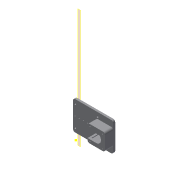
# Autodesk Inventor part: Neje_slide_y_20mmrod_upperplate
Saved by Autodesk Inventor 2019.4 (Build 234330000, 330)
## iProperties
Created: 2021-08-20
Part Number: Neje_slide_y_20mmrod_upperplate
Material: Generic
Document SubType Name: Modeling
Designer: diederichbenedict
Density: 1 g/cm^3
Appearance: Default
Mass: 53.3418 g
Surface Area: 231.662 cm^2
Volume: 53.3418 cm^3
Author: diederichbenedict
Autodesk Inventor part; units mm, degrees
ref_plane "YZ Plane" through (0, 0, 0) normal (1, 0, 0) x (0, 1, 0)
ref_plane "XZ Plane" through (0, 0, 0) normal (0, 1, 0) x (-1, 0, 0)
ref_plane "XY Plane" through (0, 0, 0) normal (0, 0, 1) x (1, 0, 0)
ref_plane "Work Plane1" through (0, 0, 0) normal (0, 0, 1) x (1, 0, 0)
sketch "Sketch1" plane through (0, 0, 0) normal (0, 0, 1) x (1, 0, 0)
  line L0 (40, 0) -> (34, 0) projected
  line L1 (40, 0) -> (40, 260) projected
  line L2 (40, 260) -> (34, 260) projected
  line L3 (34, 0) -> (34, 260) projected
  line L4 (0, 0) -> (6, 0) projected
  line L5 (6, 0) -> (6, 260) projected
  line L6 (0, 260) -> (6, 260) projected
  line L7 (0, 0) -> (0, 260) projected
  line L8 (90, 15.4736) -> (-7, 15.4736)
  line L9 (-7, 15.4736) -> (-7, 85.4736)
  line L10 (-7, 85.4736) -> (90, 85.4736)
  line L11 (90, 85.4736) -> (90, 15.4736)
  line L12 (90, 85.4736) -> (-7, 15.4736) construction
  line L13 (90, 15.4736) -> (-7, 85.4736) construction
  line L14 (14, 0) -> (26, 0) construction
  line L15 (26, 0) -> (26, 260) construction
  line L16 (14, 260) -> (26, 260) construction
  line L17 (14, 0) -> (14, 260) construction
  circle A0 centre (-2, 25.4736) radius 2.45
  circle A1 centre (-2, 75.4736) radius 2.45
  circle A2 centre (51.5, 75.4736) radius 2.45
  circle A3 centre (51.5, 25.4736) radius 2.45
  line L18 (40, 40.4736) -> (-160, 40.4736) projected
  line L19 (40, 60.4736) -> (-160, 60.4736) projected
  circle A4 centre (-2, 25.4736) radius 2.45 construction
  circle A5 centre (-2, 75.4736) radius 2.45 construction
  line L20 (-7, 67.4547) -> (-7, 33.4924) projected
  dimension "d0" = 50
  dimension "d2" = 70
  dimension "d3" = 4.9
  dimension "d4" = 4.9
  dimension "d5" = 4.9
  dimension "d6" = 4.9
  dimension "d7" = 10
  dimension "d10" = 10
  dimension "d11" = 11.5
  dimension "d17" = 25
  dimension "d20" = 0
  constraints: 12 end point, 4 centre point, 2 coincident, 2 parallel, 1 horizontal, 1 perpendicular, 1 point on line
  measures "d0" distance between parallel lines of L11 L1
  measures "d2" distance between parallel lines of L10 L8
  measures "d3" diameter of A0
  measures "d4" diameter of A1
  measures "d5" diameter of A2
  measures "d6" diameter of A3
  measures "d7" distance from line of A3.centre L8
  measures "d10" distance from line of A2.centre L10
  measures "d11" distance from line of L1 A2.centre
  measures "d17" distance between parallel lines of L18 L8
  measures "d20" horizontal distance of A2.centre A3.centre
extrude "Extrusion1" add sketch "Sketch1" along normal blind 5 contours L8 L3 L18 L1 | L1 L10 L11 L8 | L8 L5 L18 L3 | L18 L3 L19 L1 | L18 L5 L19 L3 | L8 L7 A0 L18 L5 | L19 L3 L10 L1 | L19 L5 L10 L3 | L18 L7 L19 L5 | L8 L9 L18 L7 A0 | L19 L7 A1 L10 L5 | L18 L9 L19 L7 | L19 L9 L10 L7 A1
sketch "Sketch2" plane through (0, 0, 5) normal (0, 0, 1) x (1, 0, 0)
  circle A0 centre (69, 50.4736) radius 9.2 projected
  circle A1 centre (84.5, 34.9736) radius 3 projected
  circle A2 centre (53.5, 34.9736) radius 3 projected
  circle A3 centre (53.5, 65.9736) radius 3 projected
  line L0 (89.5, 67.2664) -> (89.5, 33.6807) projected
  arc A4 (89.5, 67.2664) -> (85.7929, 70.9736) centre (69, 50.4736) ccw projected
  line L1 (52.2071, 70.9736) -> (85.7929, 70.9736) projected
  arc A5 (52.2071, 70.9736) -> (48.5, 67.2664) centre (69, 50.4736) ccw projected
  line L2 (48.5, 33.6807) -> (48.5, 67.2664) projected
  arc A6 (48.5, 33.6807) -> (52.2071, 29.9736) centre (69, 50.4736) ccw projected
  line L3 (85.7929, 29.9736) -> (52.2071, 29.9736) projected
  arc A7 (85.7929, 29.9736) -> (89.5, 33.6807) centre (69, 50.4736) ccw projected
  circle A8 centre (84.5, 34.9736) radius 3 projected
  circle A9 centre (53.5, 34.9736) radius 3 projected
  circle A10 centre (84.5, 65.9736) radius 3 projected
  circle A11 centre (69, 50.4736) radius 4 projected
  circle A12 centre (53.5, 65.9736) radius 3 projected
  point P0 (0, 0)
extrude "Extrusion2" cut sketch "Sketch2" against normal through all contours A0 | A11
sketch "Sketch3" plane through (0, 0, 5) normal (0, 0, 1) x (1, 0, 0)
  point P0 (0, 0)
sketch "Sketch4" plane through (0, 0, 5) normal (0, 0, 1) x (1, 0, 0)
  line L0 (89.5, 67.2664) -> (89.5, 33.6807) projected
  arc A0 (89.5, 67.2664) -> (85.7929, 70.9736) centre (69, 50.4736) ccw projected
  line L1 (52.2071, 70.9736) -> (85.7929, 70.9736) projected
  arc A1 (52.2071, 70.9736) -> (48.5, 67.2664) centre (69, 50.4736) ccw projected
  line L2 (48.5, 33.6807) -> (48.5, 67.2664) projected
  arc A2 (48.5, 33.6807) -> (52.2071, 29.9736) centre (69, 50.4736) ccw projected
  line L3 (85.7929, 29.9736) -> (52.2071, 29.9736) projected
  arc A3 (85.7929, 29.9736) -> (89.5, 33.6807) centre (69, 50.4736) ccw projected
  circle A4 centre (84.5, 34.9736) radius 3 projected
  circle A5 centre (53.5, 34.9736) radius 3 projected
  circle A6 centre (84.5, 65.9736) radius 3 projected
  circle A7 centre (69, 50.4736) radius 4 projected
  circle A8 centre (53.5, 65.9736) radius 3 projected
  circle A9 centre (69, 50.4736) radius 9.2
  line L4 (90, 85.4736) -> (90, 15.4736) projected
  line L5 (48, 29.9736) -> (90, 29.9736)
  line L6 (90, 29.9736) -> (90, 70.9736)
  line L7 (90, 70.9736) -> (48, 70.9736)
  line L8 (48, 29.9736) -> (90, 70.9736) construction
  line L9 (90, 29.9736) -> (48, 70.9736) construction
  arc A10 (69, 38.8858) -> (69, 62.0613) centre (69, 50.4736) ccw
  line L10 (69, 38.8858) -> (48, 38.8858)
  line L11 (48, 62.0613) -> (69, 62.0613)
  line L12 (48, 70.9736) -> (48, 62.0613)
  line L13 (48, 38.8858) -> (48, 29.9736)
  line L14 (69, 62.0613) -> (69, 46.4736)
  line L15 (69, 41.2736) -> (69, 38.8858)
  point P0 (0, 0)
  constraints: 23 end point, 4 parallel, 2 coincident, 2 horizontal, 2 midpoint, 2 point on circle, 2 vertical alignment, 1 centre point, 1 perpendicular, 1 point on line, 3 other
extrude "Extrusion3" add sketch "Sketch4" along normal blind 20 contours A0 L7 L4 L5 A3 L0 | L0 A3 L3 A2 L2 L10 A10 L11 A1 L1 A0 | A1 L2 L11 L12 L7 | L5 L13 L10 L2 A2 | A4 | A5 | A6 | A8
fillet "Fillet1" radius 5 8 edges at (90, 85.4736, 2.5) (-7, 85.4736, 2.5) (-7, 15.4736, 2.5) (90, 15.4736, 2.5) (48, 29.9736, 15) (90, 29.9736, 15) (48, 70.9736, 15) (90, 70.9736, 15)
sketch "Sketch5" plane through (0, 0, 0) normal (0, 0, -1) x (-1, 0, 0)
  line L0 (-40, 40.4736) -> (-40, 46.4736) projected
  line L1 (-40, 46.4736) -> (160, 46.4736) projected
  line L2 (160, 40.4736) -> (160, 46.4736) projected
  line L3 (-40, 40.4736) -> (160, 40.4736) projected
  line L4 (-40, 54.4736) -> (-40, 60.4736) projected
  line L5 (-40, 60.4736) -> (160, 60.4736) projected
  line L6 (160, 54.4736) -> (160, 60.4736) projected
  line L7 (-40, 54.4736) -> (160, 54.4736) projected
  circle A0 centre (12.6673, 50.4736) radius 1.45
  circle A1 centre (-27.3327, 50.4736) radius 1.45
  circle A2 centre (-7.3327, 50.4736) radius 1.45
  circle A3 centre (-47.3327, 50.4736) radius 1
  point P0 (0, 0)
  dimension "d24" = 2.9
  dimension "d25" = 2.9
  dimension "d26" = 2.9
  dimension "d27" = 4
  dimension "d28" = 4
  dimension "d29" = 4
  dimension "d30" = 20
  dimension "d31" = 20
  dimension "d39" = 2
  dimension "d40" = 4
  dimension "d41" = 20
  constraints: 4 centre point
  measures "d24" diameter of A0
  measures "d25" diameter of A1
  measures "d26" diameter of A2
  measures "d27" distance from line of A0.centre L7
  measures "d28" distance from line of A2.centre L7
  measures "d29" distance from line of A1.centre L7
  measures "d30" distance of A2.centre A0.centre
  measures "d31" distance of A1.centre A2.centre
  measures "d39" diameter of A3
  measures "d40" distance from line of A3.centre L7
  measures "d41" distance of A3.centre A1.centre
hole "Hole1" at (-12.6673, 50.4736, 0) at (47.3327, 50.4736, 0) direction (0, 0, 1) diameter 2.9 end through all counterbore diameter 7 counterbore depth 3
sketch "Sketch6" plane through (0, 0, 0) normal (0, 0, -1) x (-1, 0, 0)
  line L0 (-52.2071, 29.9736) -> (-85.7929, 29.9736) projected
  arc A0 (-52.2071, 29.9736) -> (-48.5, 33.6807) centre (-69, 50.4736) ccw projected
  line L1 (-48.5, 67.2664) -> (-48.5, 33.6807) projected
  arc A1 (-48.5, 67.2664) -> (-52.2071, 70.9736) centre (-69, 50.4736) ccw projected
  line L2 (-85.7929, 70.9736) -> (-52.2071, 70.9736) projected
  arc A2 (-85.7929, 70.9736) -> (-89.5, 67.2664) centre (-69, 50.4736) ccw projected
  line L3 (-89.5, 33.6807) -> (-89.5, 67.2664) projected
  arc A3 (-89.5, 33.6807) -> (-85.7929, 29.9736) centre (-69, 50.4736) ccw projected
  circle A4 centre (-84.5, 34.9736) radius 3 projected
  circle A5 centre (-84.5, 65.9736) radius 3 projected
  circle A6 centre (-53.5, 34.9736) radius 3 projected
  circle A7 centre (-69, 50.4736) radius 4 projected
  circle A8 centre (-53.5, 65.9736) radius 3 projected
  point P0 (0, 0)
  point P1 (-84.6331, 35.182)
hole "Hole2" at (84.5, 65.9736, 0) at (53.5, 65.9736, 0) at (53.5, 34.9736, 0) at (84.5, 34.9736, 0) direction (0, 0, 1) diameter 2.8 end through all counterbore diameter 8 counterbore depth 20
pattern_linear "Rectangular Pattern1" count 7 spacing 10 along (-1, 0, 0) of "Hole1"
equation "\"d3\" = d6"
equation "\"d4\" = d6"
equation "\"d5\" = d6"
body "Solid1"
